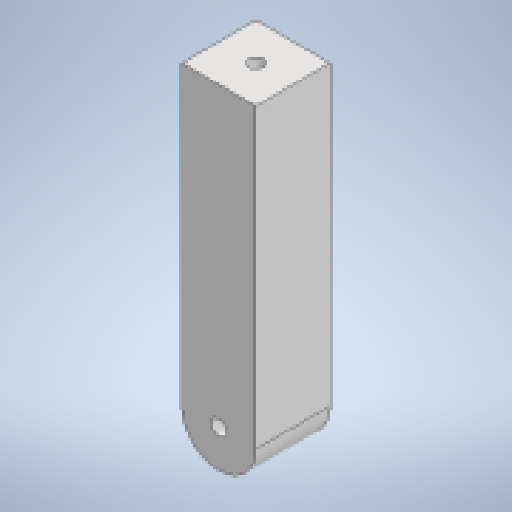
# Autodesk Inventor part: link5
Saved by Autodesk Inventor 2025.4 (Build 294407000, 407)
## iProperties
Created: 2026-03-19
Part Number: link5
Material: Generic
Document SubType Name: Modeling
Designer: dawid
Density: 1 g/cm^3
Appearance: Default
Author: dawid
Autodesk Inventor part; units mm, degrees
ref_plane "YZ Plane" through (0, 0, 0) normal (1, 0, 0) x (0, 1, 0)
ref_plane "XZ Plane" through (0, 0, 0) normal (0, 1, 0) x (-1, 0, 0)
ref_plane "XY Plane" through (0, 0, 0) normal (0, 0, 1) x (1, 0, 0)
sketch "Sketch1" plane through (0, 0, 0) normal (0, 0, 1) x (1, 0, 0)
  circle A0 centre (0, 0) radius 5
  circle A1 centre (0, 0) radius 25
  line L0 (25, 0) -> (-25, 0)
  line L1 (-25, 0) -> (-25, 200)
  line L2 (-25, 200) -> (25, 200)
  line L3 (25, 200) -> (25, 0)
  dimension "d1" = 50
  dimension "d0" = 10
  dimension "d2" = 200
  constraints: 8 end point, 2 coincident, 2 parallel, 2 vertical, 1 centre point, 1 horizontal, 1 perpendicular, 3 other
  measures "d0" diameter of A0
  measures "d2" distance of L0.end L1.end
extrude "Extrusion1" add sketch "Sketch1" along normal blind 50 contours L0 A1 A0 | A0 L0 A1 | A1 L1 L2 L3
sketch "Sketch2" plane through (-25, 200, 0) normal (0, 1, 0) x (1, 0, 0)
  line L0 (50, 0) -> (0, 0) projected
  line L1 (0, 0) -> (0, -50) projected
  point P0 (25, 0)
  point P1 (25, -25)
  dimension "d5" = 25
  dimension "d6" = 25
  measures "d5" distance from line of L0 point (25, -25)
  measures "d6" distance from line of L1 point (25, -25)
hole "Hole1" at (0, 200, 25) direction (0, -1, 0) diameter 10 depth 8 tip angle 118
body "Solid1"
